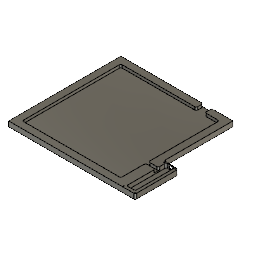
EnclosureBase_01 v13 (Autodesk Fusion 360 design; units mm, degrees)
Autodesk Fusion 360 part; units mm, degrees
note: some values were not read from the file. Set by a fixed rule: which sketch regions a step uses.
sketch "Sketch1" plane through (0, 0, 0) normal (0, 0, 1) x (1, 0, 0)
  line L0 (0, 0) -> (390, 0)
  line L1 (390, 0) -> (390, 390)
  line L2 (390, 390) -> (0, 390)
  line L3 (0, 390) -> (0, 0)
  line L4 (390, 0) -> (440, 0)
  line L5 (440, 0) -> (440, 150)
  line L6 (440, 150) -> (390, 150)
  line L7 (390, 150) -> (390, 0)
  dimension "d5" = 390
  dimension "d6" = 390
  dimension "d23" = 150
  dimension "d26" = 50
  constraint horizontal L0
  constraint vertical L1
  constraint horizontal L2
  constraint vertical L3
  constraint coincident L0.start L3.end
  constraint horizontal L4
  constraint vertical L5
  constraint horizontal L6
  constraint vertical L7
  measures "d5" distance of L0.start L2.end
  measures "d6" distance of L0.start L0.end
  measures "d23" distance of L4 L6
  measures "d26" distance of L0.end L4.end
extrude "Extrude1" add sketch "Sketch1" along normal blind 18
fillet "Fillet2" radius 5 3 edges at (440, 0, 9) (440, 150, 9) (390, 150, 9)
sketch "Sketch4" plane through (0, 0, 18) normal (0, 0, 1) x (-1, 0, 0)
  arc A0 (-440, -145) -> (-435, -150) centre (-435, -145) ccw
  line L0 (-435, -150) -> (-395, -150)
  arc A1 (-390, -155) -> (-395, -150) centre (-395, -155) ccw
  line L1 (-390, -155) -> (-390, -390)
  line L2 (-390, -390) -> (0, -390)
  line L3 (0, -390) -> (0, 0)
  line L4 (0, 0) -> (-435, 0)
  arc A2 (-435, 0) -> (-440, -5) centre (-435, -5) ccw
  line L5 (-440, -5) -> (-440, -145)
  line L6 (-400, -148) -> (-430, -148)
  line L7 (-430, -148) -> (-430, -10)
  line L8 (-430, -10) -> (-400, -10)
  line L9 (-400, -10) -> (-400, -148)
  point P0 (-395, -145)
  point P1 (-435, -145)
  point P2 (-435, -5)
  point P3 (-395, -5)
  dimension "d28" = 10
  dimension "d29" = 10
  dimension "d30" = 10
  dimension "d38" = 2
  dimension "d50" = 5
  dimension "d51" = 5
  dimension "d52" = 5
  dimension "d53" = 5
  dimension "d54" = 5
  dimension "d55" = 45
  dimension "d59" = 45
  constraint horizontal L6
  constraint vertical L7
  constraint horizontal L8
  constraint vertical L9
  constraint coincident P1 A0.centre
  constraint coincident P2 A2.centre
  measures "d28" distance of L5 L7
  measures "d29" distance of L1 L9
  measures "d30" distance of L4 L8
  measures "d38" distance of L0 L6
  measures "d50" distance of L4 P3
  measures "d51" distance of L4.end P2
  measures "d52" distance of L5 P2
  measures "d53" distance of L5 P1
  measures "d54" distance of L0 P0
  measures "d55" distance of L5 P0
  measures "d59" distance of L5 P3
extrude "Extrude4" cut sketch "Sketch4" against normal blind 14.4 contours L6 L7 L8 L9
fillet "Fillet3" radius 5 4 edges at (400, 10, 10.8) (430, 10, 10.8) (400, 148, 10.8) (430, 148, 10.8)
sketch "Sketch5" plane through (0, 0, 18) normal (0, 0, 1) x (-1, 0, 0)
  line L0 (-400, -15) -> (-400, -143)
  arc A0 (-390, -155) -> (-395, -150) centre (-395, -155) ccw
  line L1 (-390, -155) -> (-390, -390)
  line L2 (-390, -390) -> (0, -390)
  line L3 (0, -390) -> (0, 0)
  line L4 (0, 0) -> (-435, 0)
  arc A1 (-435, 0) -> (-440, -5) centre (-435, -5) ccw
  line L5 (-440, -5) -> (-440, -145)
  arc A2 (-440, -145) -> (-435, -150) centre (-435, -145) ccw
  line L6 (-435, -150) -> (-395, -150)
  line L7 (-430, -143) -> (-430, -15)
  arc A3 (-425, -10) -> (-430, -15) centre (-425, -15) ccw
  line L8 (-425, -10) -> (-405, -10)
  arc A4 (-400, -15) -> (-405, -10) centre (-405, -15) ccw
  line L9 (-24, -366) -> (-366, -366)
  line L10 (-366, -366) -> (-366, -24)
  line L11 (-366, -24) -> (-24, -24)
  line L12 (-24, -24) -> (-24, -366)
  line L13 (-405, -148) -> (-425, -148)
  arc A5 (-405, -148) -> (-400, -143) centre (-405, -143) ccw
  arc A6 (-430, -143) -> (-425, -148) centre (-425, -143) ccw
  line L14 (-316, -366) -> (-316, -390)
  line L15 (-316, -390) -> (-286, -390)
  line L16 (-286, -390) -> (-286, -366)
  line L17 (-366, -120) -> (-400, -120)
  line L18 (-400, -120) -> (-400, -110)
  line L19 (-400, -110) -> (-366, -110)
  line L20 (-366, -110) -> (-366, -120)
  dimension "d34" = 342
  dimension "d35" = 342
  dimension "d36" = 24
  dimension "d37" = 24
  dimension "d41" = 50
  dimension "d42" = 30
  dimension "d60" = 30
  dimension "d61" = 10
  constraint horizontal L9
  constraint vertical L10
  constraint horizontal L11
  constraint vertical L12
  constraint vertical L14
  constraint horizontal L15
  constraint vertical L16
  constraint coincident L2 L14.end
  constraint coincident L9 L16.end
  constraint coincident L9 L14.start
  constraint horizontal L17
  constraint vertical L18
  constraint horizontal L19
  constraint vertical L20
  constraint coincident L0 L18.end
  constraint coincident L10 L17.start
  measures "d34" distance of L10 L12
  measures "d35" distance of L9 L11
  measures "d36" distance of L3 L12
  measures "d37" distance of L2 L9
  measures "d41" distance of L10 L14
  measures "d42" distance of L14 L16
  measures "d60" distance of L6 L17
  measures "d61" distance of L17 L19
extrude "Extrude5" cut sketch "Sketch5" against normal blind 10 contours L0 L10 L17 L18 L19 L20 | L9 L10 L11 L12 L20 | L2 L9 L14 L15 L16
fillet "Fillet4" radius 5 8 edges at (24, 366, 13) (286, 366, 13) (24, 24, 13) (366, 24, 13) (366, 366, 13) (316, 366, 13) (316, 390, 13) (286, 390, 13)
fillet "Fillet4" radius 5 4 edges at (366, 120, 13) (400, 120, 13) (366, 110, 13) (400, 110, 13)
sketch "Sketch6" plane through (0, 150, 0) normal (0, 1, 0) x (-1, 0, 0)
  line L0 (-395, 0) -> (-395, 18)
  line L1 (-435, 18) -> (-435, 0)
  line L2 (-435, 0) -> (-395, 0)
  line L3 (-440, 18) -> (-440, 0)
  line L4 (-395, 18) -> (-435, 18)
  point P0 (-415, 10)
  dimension "d45" = 25
  dimension "d46" = 10
  measures "d45" distance of P0 L3
  measures "d46" distance of L2 P0
hole "Hole1" at (415, 150, 10) direction (0, -1, 0) diameter 10 depth 2 tip angle 118
hole "Hole2" at (395, 5, 18) at (435, 5, 18) at (435, 145, 18) at (395, 145, 18) direction (0, 0, -1) diameter 3 depth 10 tip angle 118
equation "b = 350 mm"
equation "d = 350 mm"
equation "t_base = 18 mm"
equation "a_ramme = 20 mm"
equation "d5 = d + 2 * a_ramme"
equation "d6 = b + 2 * a_ramme"
equation "d7 = t_base"
equation "t = 4 mm"
equation "a_outlet = 30 mm"
equation "d23 = d_utilites"
equation "b_utilities = 50 mm"
equation "d_utilites = 150 mm"
equation "d26 = b_utilities"
equation "d31 = -t_base * 0.8"
equation "d34 = b - 2 * t"
equation "d35 = d - 2 * t"
equation "d36 = a_ramme + t"
equation "d37 = a_ramme + t"
equation "d42 = a_outlet"
